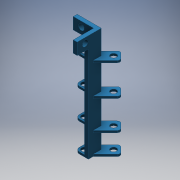
# Autodesk Inventor part: VerticalConnector
Saved by Autodesk Inventor 2016 (Build 200138000, 138)
## iProperties
Created: 2015-06-01
Part Number: VerticalConnector
Material: Generic
Document SubType Name: Modeling
Designer: Erin
Density: 1 g/cm^3
Appearance: Default
Author: Erin
Autodesk Inventor part; units mm, degrees
sketch "Sketch1" plane through (0, 0, 0) normal (0, 0, 1) x (1, 0, 0)
  line L0 (-0.2363, 14.3955) -> (15.4637, 14.3955)
  line L1 (15.4637, 14.3955) -> (15.4637, 17.3955)
  line L2 (15.4637, 17.3955) -> (-0.2363, 17.3955)
  line L3 (-0.2363, 17.3955) -> (-0.2363, 14.3955)
  line L4 (15.4637, 14.3955) -> (18.4637, 14.3955)
  line L5 (18.4637, 14.3955) -> (18.4637, -1.3045)
  line L6 (18.4637, -1.3045) -> (15.4637, -1.3045)
  line L7 (15.4637, -1.3045) -> (15.4637, 14.3955)
  line L8 (15.4637, 14.3955) -> (18.4637, 14.3955)
  line L9 (18.4637, 14.3955) -> (18.4637, 17.3955)
  line L10 (18.4637, 17.3955) -> (15.4637, 17.3955)
  line L11 (15.4637, 17.3955) -> (15.4637, 14.3955)
  circle A0 centre (11.9637, 10.8955) radius 2.25
  line L12 (15.4637, 14.3955) -> (8.4637, 14.3955)
  line L13 (8.4637, 14.3955) -> (8.4637, 7.3955)
  line L14 (8.4637, 7.3955) -> (15.4637, 7.3955)
  line L15 (15.4637, 7.3955) -> (15.4637, 14.3955)
  point P0 (0, 0)
  point P1 (11.9637, 7.3955)
  point P2 (8.4637, 10.8955)
  dimension "d2" = 3
  dimension "d3" = 3
  dimension "d9" = 4.5
  dimension "d46" = 7
  dimension "d47" = 7
  dimension "d48" = 15.7
  dimension "d49" = 15.7
  constraints: 32 end point, 8 parallel, 4 horizontal, 4 perpendicular, 2 midpoint, 2 point on line, 1 centre point, 1 horizontal alignment, 1 vertical alignment
  measures "d2" distance of L1.end L0.end
  measures "d3" distance of L5.end L6.end
  measures "d9" diameter of A0
  measures "d46" distance of L14.end L13.end
  measures "d47" distance of L13.end L12.end
  measures "d48" distance of L4.end L5.end
  measures "d49" distance of L1.end L2.end
extrude "Extrusion1" add sketch "Sketch1" along normal blind 83 contours L3 L2 L1 L0 | L1 L10 L9 L4 | L4 L5 L6 L7
extrude "Extrusion2" add sketch "Sketch1" along normal blind 1.5 contours L0 L7 L14 L13
fillet "Fillet1" radius 3 1 edges at (8.4637, 7.3955, 0.75)
sketch "Sketch3" plane through (-0.2363, 14.3955, 83) normal (0, -1, 0) x (1, 0, 0)
  line L0 (15.7, 0) -> (15.7, -81.5) projected
  line L1 (0, 0) -> (15.7, 0) projected
  line L2 (0, -83) -> (0, 0) projected
  circle A0 centre (6.25, -4) radius 2.25
  line L3 (18.7, -83) -> (0, -83) projected
  line L4 (0, 0) -> (15.7, 0) projected
  line L5 (18.7, 0) -> (0, 0) projected
  line L6 (12.5, 0) -> (12.5, -83) construction
  line L7 (0, -83) -> (0, 0) projected
  line L8 (12.5, 0) -> (0, 0)
  line L9 (0, -83) -> (8.7, -83) projected
  line L10 (8.7, -81.5) -> (15.7, -81.5) projected
  line L11 (8.7, -83) -> (8.7, -81.5) projected
  point P0 (0.2363, -83)
  point P1 (1.7, -20)
  point P2 (6.25, 0)
  dimension "d12" = 4.5
  dimension "d13" = 4
  dimension "d24" = 12.5
  constraints: 4 end point, 1 centre point, 1 horizontal, 1 midpoint, 1 point on line, 1 vertical, 1 vertical alignment, 2 other
  measures "d12" diameter of A0
  measures "d13" distance from line of A0.centre L1
  measures "d24" distance between parallel lines of L2 L6
sketch "Sketch4" plane through (15.4637, -1.3045, 83) normal (-1, 0, 0) x (0, 0, 1)
  line L0 (-83, 0) -> (0, 0) projected
  line L1 (0, 15.7) -> (0, 0) projected
  line L2 (0, 15.7) -> (-81.5, 15.7) projected
  circle A0 centre (-4, 6.25) radius 2.25
  line L3 (0, 15.7) -> (0, 0) projected
  line L4 (-83, 0) -> (-83, 18.7) projected
  line L5 (0, 15.7) -> (-81.5, 15.7) projected
  line L6 (0, 12.5) -> (-83, 12.5) construction
  line L7 (0, 12.5) -> (0, 0)
  line L8 (-83, 8.7) -> (-83, 0) projected
  line L9 (-81.5, 15.7) -> (-81.5, 8.7) projected
  line L10 (-81.5, 8.7) -> (-83, 8.7) projected
  point P0 (-83, 1.3045)
  point P1 (-20, 1.7)
  point P2 (0, 6.25)
  point P3 (-83, 15.7)
  dimension "d14" = 4.5
  dimension "d15" = 4
  dimension "d25" = 12.5
  constraints: 4 end point, 1 centre point, 1 collinear, 1 horizontal, 1 horizontal alignment, 1 midpoint, 1 point on line, 2 other
  measures "d14" diameter of A0
  measures "d15" distance from line of A0.centre L1
  measures "d25" distance between parallel lines of L6 L0
extrude "Extrusion4" cut sketch "Sketch3" against normal blind 5 contours A0
extrude "Extrusion5" cut sketch "Sketch4" against normal blind 5 contours A0
sketch "Sketch5" plane through (0, 0, 0) normal (0, 0, 1) x (1, 0, 0)
  line L0 (29.2522, 21.8201) -> (22.8883, 28.184)
  line L1 (22.8883, 28.184) -> (12.2817, 17.5774)
  line L2 (12.2817, 17.5774) -> (18.6456, 11.2135)
  line L3 (18.6456, 11.2135) -> (29.2522, 21.8201)
  line L4 (26.0703, 25.0021) -> (15.4637, 14.3955) construction
  line L5 (23.9489, 16.5168) -> (17.585, 22.8807) construction
  line L6 (15.4637, -1.3045) -> (15.4637, 14.3955) projected
  line L7 (15.4637, 17.3955) -> (-0.2363, 17.3955) projected
  line L8 (18.4637, 14.3955) -> (18.4637, -1.3045) projected
  line L9 (18.4637, 14.3955) -> (18.4637, 17.3955) projected
  line L10 (18.4637, 17.3955) -> (15.4637, 17.3955) projected
  circle A0 centre (23.2418, 22.1736) radius 2.25
  line L11 (18.0923, 10.6601) -> (18.6456, 11.2135)
  line L12 (18.6456, 11.2135) -> (12.2817, 17.5774)
  line L13 (12.2817, 17.5774) -> (11.7283, 17.0241)
  line L14 (11.7283, 17.0241) -> (18.0923, 10.6601)
  point P0 (0, 0)
  dimension "d29" = 9
  dimension "d30" = 4.5
  dimension "d31" = 4
  dimension "d32" = 15
  dimension "d56" = 9
  constraints: 20 end point, 5 equal length, 4 midpoint, 2 collinear, 2 perpendicular, 2 point on line, 1 centre point
  measures "d29" distance of L1.end L2.end
  measures "d30" diameter of A0
  measures "d31" distance from line of A0.centre L0
  measures "d32" distance of L2.end L0.start
  measures "d56" distance of L12.end L11.end
extrude "Extrusion6" add sketch "Sketch5" along normal blind 1.5
fillet "Fillet2" radius 2 2 edges at (22.8883, 28.184, 0.75) (29.2522, 21.8201, 0.75)
ref_plane "Work Plane2" through (0, 0, 74) normal (0, 0, 1) x (1, 0, 0)
sketch "Sketch6" plane through (0, 0, 74) normal (0, 0, 1) x (1, 0, 0)
  line L0 (18.4637, -1.3045) -> (18.4637, 17.3955)
  line L1 (18.4637, 17.3955) -> (-0.2363, 17.3955)
  line L2 (-0.2363, 17.3955) -> (-0.2363, 14.3955)
  line L3 (15.4637, -1.3045) -> (18.4637, -1.3045)
  line L4 (-0.2363, 17.3955) -> (-0.2363, 14.3955) projected
  line L5 (-0.2363, 17.3955) -> (8.4637, 17.3955)
  line L6 (8.4637, 17.3955) -> (8.4637, 14.3955)
  line L7 (8.4637, 14.3955) -> (-0.2363, 14.3955)
  line L8 (-0.2363, 14.3955) -> (-0.2363, 17.3955)
  line L9 (18.4637, -1.3045) -> (15.4637, -1.3045)
  line L10 (15.4637, -1.3045) -> (15.4637, 7.3955)
  line L11 (15.4637, 7.3955) -> (18.4637, 7.3955)
  line L12 (18.4637, 7.3955) -> (18.4637, -1.3045)
  point P0 (0, 0)
  dimension "d45" = 8.7
  dimension "d50" = 7
  dimension "d51" = 7
  constraints: 24 end point, 4 parallel, 2 horizontal, 2 perpendicular
  measures "d45" distance between parallel lines of L6 L2
  measures "d50" distance between parallel lines of L7 L11
  measures "d51" distance between parallel lines of L10 L6
extrude "Extrusion7" cut sketch "Sketch6" against normal blind 74
ref_plane "Work Plane3" through (0, 0, 43) normal (0, 0, 1) x (1, 0, 0)
ref_plane "Work Plane5" through (0, 0, 39) normal (0, 0, 1) x (1, 0, 0)
sketch "Sketch9" plane through (0, 0, 39) normal (0, 0, 1) x (1, 0, 0)
  line L0 (18.4637, 7.3955) -> (11.4637, 7.3955) projected
  arc A0 (8.4637, 10.3955) -> (11.4637, 7.3955) centre (11.4637, 10.3955) ccw projected
  line L1 (8.4637, 10.3955) -> (8.4637, 17.3955) projected
  line L2 (12.0997, 17.3955) -> (8.4637, 17.3955) projected
  line L3 (21.4741, 26.7698) -> (12.0997, 17.3955) projected
  arc A1 (24.3025, 26.7698) -> (21.4741, 26.7698) centre (22.8883, 25.3556) ccw projected
  line L4 (27.838, 23.2343) -> (24.3025, 26.7698) projected
  arc A2 (27.838, 20.4059) -> (27.838, 23.2343) centre (26.4238, 21.8201) ccw projected
  line L5 (18.4637, 11.0315) -> (27.838, 20.4059) projected
  line L6 (18.4637, 7.3955) -> (18.4637, 11.0315) projected
  circle A3 centre (23.2418, 22.1736) radius 2.25 projected
  circle A4 centre (11.9637, 10.8955) radius 2.25 projected
  line L7 (12.0997, 17.3955) -> (16.4707, 15.4026)
  line L8 (16.4707, 15.4026) -> (18.4637, 11.0315)
  point P0 (0, 0)
  constraints: 4 end point
extrude "Extrusion9" add sketch "Sketch9" along normal blind 1.5 contours L8 L7 L3 A1 L4 A2 L5
ref_plane "Work Plane6" through (0, 0, 16) normal (0, 0, 1) x (1, 0, 0)
sketch "Sketch10" plane through (0, 0, 16) normal (0, 0, 1) x (1, 0, 0)
  line L0 (18.4637, 7.3955) -> (11.4637, 7.3955) projected
  arc A0 (8.4637, 10.3955) -> (11.4637, 7.3955) centre (11.4637, 10.3955) ccw projected
  line L1 (8.4637, 10.3955) -> (8.4637, 17.3955) projected
  line L2 (12.0997, 17.3955) -> (8.4637, 17.3955) projected
  line L3 (21.4741, 26.7698) -> (12.0997, 17.3955) projected
  arc A1 (24.3025, 26.7698) -> (21.4741, 26.7698) centre (22.8883, 25.3556) ccw projected
  line L4 (27.838, 23.2343) -> (24.3025, 26.7698) projected
  arc A2 (27.838, 20.4059) -> (27.838, 23.2343) centre (26.4238, 21.8201) ccw projected
  line L5 (18.4637, 11.0315) -> (27.838, 20.4059) projected
  line L6 (18.4637, 7.3955) -> (18.4637, 11.0315) projected
  circle A3 centre (23.2418, 22.1736) radius 2.25 projected
  circle A4 centre (11.9637, 10.8955) radius 2.25 projected
  line L7 (12.0997, 17.3955) -> (18.4637, 17.3955) projected
  line L8 (12.0997, 17.3955) -> (16.7869, 15.7187)
  line L9 (18.4637, 17.3955) -> (18.4637, 11.0315) projected
  line L10 (16.7869, 15.7187) -> (18.4637, 11.0315)
  point P0 (0, 0)
  constraints: 4 end point
extrude "Extrusion10" add sketch "Sketch10" along normal blind 1.5 contours L9 L7 L3 A1 L4 A2 L5
pattern_linear "Rectangular Pattern2" count 4 spacing 22 along (0, 0, 1) of "Extrusion2", "Fillet1"
ref_plane "Work Plane7" through (0, 0, 63) normal (0, 0, 1) x (1, 0, 0)
sketch "Sketch11" plane through (0, 0, 63) normal (0, 0, 1) x (1, 0, 0)
  arc A0 (27.838, 20.4059) -> (27.838, 23.2343) centre (26.4238, 21.8201) ccw projected
  line L0 (18.4637, 7.3955) -> (11.4637, 7.3955) projected
  arc A1 (8.4637, 10.3955) -> (11.4637, 7.3955) centre (11.4637, 10.3955) ccw projected
  line L1 (8.4637, 10.3955) -> (8.4637, 17.3955) projected
  line L2 (12.0997, 17.3955) -> (8.4637, 17.3955) projected
  line L3 (21.4741, 26.7698) -> (12.0997, 17.3955) projected
  arc A2 (24.3025, 26.7698) -> (21.4741, 26.7698) centre (22.8883, 25.3556) ccw projected
  line L4 (27.838, 23.2343) -> (24.3025, 26.7698) projected
  arc A3 (27.838, 20.4059) -> (27.838, 23.2343) centre (26.4238, 21.8201) ccw projected
  line L5 (18.4637, 11.0315) -> (27.838, 20.4059) projected
  line L6 (18.4637, 7.3955) -> (18.4637, 11.0315) projected
  circle A4 centre (23.2418, 22.1736) radius 2.25 projected
  circle A5 centre (11.9637, 10.8955) radius 2.25 projected
  line L7 (18.4637, 11.0315) -> (16.7869, 15.7187)
  line L8 (16.7869, 15.7187) -> (12.0997, 17.3955)
  point P0 (0, 0)
  constraints: 4 end point
extrude "Extrusion11" add sketch "Sketch11" along normal blind 1.5 contours L5 L7 L8 L3 A2 L4 A0
body "Solid1"
